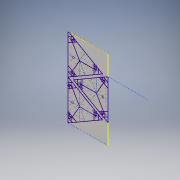
# Autodesk Inventor part: design(60,60,60)_3frames
Saved by Autodesk Inventor 2016 (Build 200138000, 138)
## iProperties
Created: 2016-02-28
Part Number: design(60,60,60)_3frames
Material: Generic
Document SubType Name: Modeling
Designer: Raghu Velagala
Density: 1 g/cm^3
Appearance: Default
Author: Raghu Velagala
Autodesk Inventor part; units mm, degrees
ref_plane "YZ Plane" through (0, 0, 0) normal (1, 0, 0) x (0, 1, 0)
ref_plane "XZ Plane" through (0, 0, 0) normal (0, 1, 0) x (-1, 0, 0)
ref_plane "XY Plane" through (0, 0, 0) normal (0, 0, 1) x (1, 0, 0)
sketch "Sketch1" plane through (0, 0, 0) normal (0, 0, 1) x (1, 0, 0)
  line L0 (0, 0) -> (304.8, 0)
  line L1 (304.8, 0) -> (304.8, 609.6)
  line L2 (304.8, 609.6) -> (0, 609.6)
  line L3 (0, 609.6) -> (0, 0)
  dimension "d4" = 609.6
  dimension "d5" = 304.8
  constraints: 8 end point, 2 parallel, 1 horizontal, 1 perpendicular
  measures "d4" distance of L0.end L1.end
  measures "d5" distance of L1.end L2.end
extrude "Extrusion1" add sketch "Sketch1" along normal blind 1.6002
sketch "3 frames" plane through (0, 0, 1.6002) normal (0, 0, 1) x (1, 0, 0)
  line L0 (0, 609.6) -> (0, 0) projected
  line L1 (0, 609.6) -> (263.9645, 457.2)
  line L2 (0, 609.6) -> (304.8, 609.6) construction
  line L3 (263.9645, 457.2) -> (0, 304.8)
  line L4 (0, 0) -> (263.9645, 152.4)
  line L5 (0, 0) -> (304.8, 0) construction
  line L6 (263.9645, 152.4) -> (0, 304.8)
  line L7 (197.9734, 419.1) -> (197.9734, 495.3)
  line L8 (304.8, 0) -> (304.8, 609.6) projected
  line L9 (304.8, 0) -> (304.8, 609.6) projected
  line L10 (304.8, 459.0878) -> (40.8355, 306.6878)
  line L11 (304.8, 459.0878) -> (609.6, 459.0878) construction
  line L12 (40.8355, 306.6878) -> (304.8, 154.2878)
  line L13 (65.9911, 38.1) -> (0, 76.2)
  line L14 (197.9734, 114.3) -> (197.9734, 190.5)
  line L15 (0, 228.6) -> (65.9911, 266.7)
  line L16 (238.8089, 192.3878) -> (304.8, 230.4878)
  line L17 (238.8089, 420.9878) -> (304.8, 382.8878)
  line L18 (106.8266, 268.5878) -> (106.8266, 344.7878)
  line L19 (65.9911, 342.9) -> (0, 381)
  line L20 (0, 533.4) -> (65.9911, 571.5)
  line L21 (271.8044, 440.0378) -> (304.8, 420.9878)
  line L22 (256.5553, 417.5255) -> (265.1553, 432.4212)
  line L23 (100.9518, 285.6878) -> (83.7518, 285.6878)
  line L24 (256.5553, 195.8501) -> (265.1553, 180.9545)
  line L25 (11.8716, 242.2377) -> (3.2716, 257.1333)
  line L26 (203.8482, 173.4) -> (221.0482, 173.4)
  line L27 (11.8716, 62.5623) -> (3.2716, 47.6667)
  line L28 (203.8482, 478.2) -> (221.0482, 478.2)
  line L29 (48.2447, 568.0377) -> (39.6447, 582.9333)
  line L30 (48.2447, 346.3623) -> (39.6447, 331.4667)
  line L31 (230.969, 133.35) -> (230.969, 171.45)
  line L32 (0, 266.7) -> (32.9956, 285.75)
  line L33 (32.9956, 19.05) -> (0, 38.1)
  line L34 (271.8044, 173.3378) -> (304.8, 192.3878)
  line L35 (73.831, 287.6378) -> (73.831, 325.7378)
  line L36 (0, 342.9) -> (32.9956, 323.85)
  line L37 (230.969, 438.15) -> (230.969, 476.25)
  line L38 (0, 571.5) -> (32.9956, 590.55)
  line L39 (7.5716, 55.1145) -> (25.7582, 44.6145)
  line L40 (212.4482, 173.4) -> (212.4482, 152.4)
  line L41 (7.5716, 249.6855) -> (25.7582, 260.1855)
  line L42 (260.8553, 188.4023) -> (279.0418, 198.9023)
  line L43 (92.3518, 285.6878) -> (92.3518, 306.6878)
  line L44 (260.8553, 424.9733) -> (279.0418, 414.4733)
  line L45 (43.9447, 338.9145) -> (25.7582, 349.4145)
  line L46 (212.4482, 478.2) -> (212.4482, 457.2)
  line L47 (43.9447, 575.4855) -> (25.7582, 564.9855)
  line L48 (0, 304.8) -> (0, 0)
  line L49 (0, 152.4) -> (263.9645, 152.4) construction
  line L50 (0, 304.8) -> (131.9823, 76.2) construction
  line L51 (0, 0) -> (131.9823, 228.6) construction
  line L52 (87.9882, 152.4) -> (87.9882, 45.6952) construction
  line L53 (87.9882, 152.4) -> (87.9882, 254) construction
  line L54 (87.9882, 152.4) -> (25.7582, 260.1855)
  line L55 (87.9882, 152.4) -> (25.7582, 44.6145)
  line L56 (87.9882, 152.4) -> (212.4482, 152.4)
  line L57 (304.8, 459.0878) -> (304.8, 154.2878)
  line L58 (304.8, 459.0878) -> (172.8177, 230.4878) construction
  line L59 (172.8177, 382.8878) -> (304.8, 154.2878) construction
  line L60 (304.8, 306.6878) -> (40.8355, 306.6878) construction
  line L61 (216.8118, 306.6878) -> (216.8118, 408.2878) construction
  line L62 (216.8118, 306.6878) -> (279.0418, 414.4733)
  line L63 (216.8118, 306.6878) -> (279.0418, 198.9023)
  line L64 (216.8118, 306.6878) -> (92.3518, 306.6878)
  line L65 (0, 304.8) -> (0, 609.6)
  line L66 (0, 304.8) -> (131.9823, 533.4) construction
  line L67 (304.8, 609.6) -> (0, 609.6) projected
  line L68 (0, 609.6) -> (131.9823, 381) construction
  line L69 (0, 457.2) -> (263.9645, 457.2) construction
  line L70 (87.9882, 457.2) -> (87.9882, 355.6) construction
  line L71 (87.9882, 457.2) -> (25.7582, 564.9855)
  line L72 (87.9882, 457.2) -> (25.7582, 349.4145)
  line L73 (87.9882, 457.2) -> (212.4482, 457.2)
  point P0 (15.3659, 50.6145)
  point P1 (212.4482, 164.4)
  point P2 (15.3659, 254.1855)
  point P3 (268.6495, 192.9023)
  point P4 (92.3518, 294.6878)
  point P5 (268.6495, 420.4733)
  point P6 (36.1505, 343.4145)
  point P7 (212.4482, 469.2)
  point P8 (36.1505, 570.9855)
  dimension "d7" = 30
  dimension "d9" = 60
  dimension "d11" = 30
  dimension "d20" = 60
  dimension "d27" = 304.8
  dimension "d28" = 150
  dimension "d29" = 304.8
  dimension "d30" = 60
  dimension "d31" = 76.2
  dimension "d32" = 76.2
  dimension "d33" = 76.2
  dimension "d34" = 76.2
  dimension "d35" = 76.2
  dimension "d36" = 76.2
  dimension "d38" = 76.2
  dimension "d39" = 76.2
  dimension "d40" = 76.2
  dimension "d81" = 17.2
  dimension "d82" = 154.2878
  dimension "d83" = 17.2
  dimension "d84" = 17.2
  dimension "d85" = 17.2
  dimension "d86" = 17.2
  dimension "d87" = 17.2
  dimension "d88" = 17.2
  dimension "d89" = 17.2
  dimension "d90" = 17.2
  dimension "d91" = 38.1
  dimension "d118" = 38.1
  dimension "d119" = 38.1
  dimension "d120" = 38.1
  dimension "d121" = 38.1
  dimension "d122" = 38.1
  dimension "d123" = 38.1
  dimension "d124" = 38.1
  dimension "d125" = 38.1
  dimension "d155" = 21
  dimension "d157" = 9
  dimension "d158" = 21
  dimension "d159" = 9
  dimension "d160" = 21
  dimension "d164" = 9
  dimension "d165" = 21
  dimension "d166" = 9
  dimension "d167" = 21
  dimension "d168" = 9
  dimension "d169" = 21
  dimension "d170" = 9
  dimension "d171" = 21
  dimension "d172" = 9
  dimension "d173" = 21
  dimension "d174" = 9
  dimension "d175" = 21
  dimension "d176" = 9
  dimension "d214" = 150
  dimension "d215" = 124.46
  dimension "d216" = 30
  dimension "d217" = 124.46
  dimension "d218" = 124.46
  dimension "d219" = 90
  dimension "d220" = 124.46
  dimension "d221" = 124.46
  dimension "d222" = 124.46
  dimension "d224" = 30
  constraints: 140 end point, 47 point on line, 27 coincident, 18 midpoint, 18 parallel, 17 perpendicular, 4 vertical, 3 equal length, 3 horizontal, 1 collinear, 9 other
  measures "d7" angle of L1 L2
  measures "d9" angle of L1 L3
  measures "d11" angle of L5 L4
  measures "d20" angle of L4 L6
  measures "d27" distance of L10.start L10.end
  measures "d28" angle of L10 L11
  measures "d29" distance of L10.end L12.end
  measures "d30" angle of L12 L10
  measures "d31" distance of L20.start L20.end
  measures "d32" distance of L7.start L7.end
  measures "d33" distance of L19.start L19.end
  measures "d34" distance of L15.start L15.end
  measures "d35" distance of L14.start L14.end
  measures "d36" distance of L18.start L18.end
  measures "d38" distance of L17.start L17.end
  measures "d39" distance of L16.start L16.end
  measures "d40" distance of L13.start L13.end
  measures "d81" distance of L22.start L22.end
  measures "d82" distance of L5.end L12.end
  measures "d83" distance of L23.start L23.end
  measures "d84" distance of L24.start L24.end
  measures "d85" distance of L25.start L25.end
  measures "d86" distance of L26.start L26.end
  measures "d87" distance of L27.start L27.end
  measures "d88" distance of L28.start L28.end
  measures "d89" distance of L29.start L29.end
  measures "d90" distance of L30.start L30.end
  measures "d91" distance of L21.start L21.end
  measures "d118" distance of L31.start L31.end
  measures "d119" distance of L33.start L33.end
  measures "d120" distance of L32.start L32.end
  measures "d121" distance of L34.start L34.end
  measures "d122" distance of L35.start L35.end
  measures "d123" distance of L37.start L37.end
  measures "d124" distance of L36.start L36.end
  measures "d125" distance of L38.start L38.end
  measures "d155" distance of L39.start L39.end
  measures "d157" distance of L39.start point (15.366, 50.614)
  measures "d158" distance of L40.start L40.end
  measures "d159" distance of L40.start point (212.448, 164.4)
  measures "d160" distance of L41.start L41.end
  measures "d164" distance of L41.start point (15.366, 254.186)
  measures "d165" distance of L42.start L42.end
  measures "d166" distance of L42.start point (268.65, 192.902)
  measures "d167" distance of L43.start L43.end
  measures "d168" distance of L43.start point (92.352, 294.688)
  measures "d169" distance of L44.start L44.end
  measures "d170" distance of L44.start point (268.65, 420.473)
  measures "d171" distance of L45.start L45.end
  measures "d172" distance of L45.start point (36.15, 343.414)
  measures "d173" distance of L46.start L46.end
  measures "d174" distance of L46.start point (212.448, 469.2)
  measures "d175" distance of L47.start L47.end
  measures "d176" distance of L47.start point (36.15, 570.986)
  measures "d214" angle of L54 L52
  measures "d215" distance of L52.start L54.end
  measures "d216" angle of L55 L52
  measures "d217" distance of L52.start L55.end
  measures "d218" distance of L52.start L56.end
  measures "d219" angle of L56 L52
  measures "d220" distance of L61.start L62.end
  measures "d221" distance of L61.start L63.end
  measures "d222" distance of L61.start L64.end
  measures "d224" angle of L62 L61
sketch "Holes" plane through (0, 0, 1.6002) normal (0, 0, 1) x (1, 0, 0)
  line L0 (182.8074, 366.1889) -> (205.8074, 366.1889)
  line L1 (205.8074, 366.1889) -> (205.8074, 308.1889)
  line L2 (205.8074, 308.1889) -> (182.8074, 308.1889)
  line L3 (182.8074, 308.1889) -> (182.8074, 366.1889)
  line L4 (102.5125, 80.9532) -> (79.5125, 80.9532)
  line L5 (79.5125, 80.9532) -> (79.5125, 138.9532)
  line L6 (79.5125, 138.9532) -> (102.5125, 138.9532)
  line L7 (102.5125, 138.9532) -> (102.5125, 80.9532)
  line L8 (119.975, 391.4712) -> (96.975, 391.4712)
  line L9 (96.975, 391.4712) -> (96.975, 449.4712)
  line L10 (96.975, 449.4712) -> (119.975, 449.4712)
  line L11 (119.975, 449.4712) -> (119.975, 391.4712)
  line L12 (169.2482, 365.9) -> (218.2482, 365.9)
  line L13 (218.2482, 365.9) -> (218.2482, 307.9)
  line L14 (218.2482, 307.9) -> (169.2482, 307.9)
  line L15 (169.2482, 307.9) -> (169.2482, 365.9)
  line L16 (65.4689, 138.9625) -> (114.4689, 138.9625)
  line L17 (114.4689, 138.9625) -> (114.4689, 80.9625)
  line L18 (114.4689, 80.9625) -> (65.4689, 80.9625)
  line L19 (65.4689, 80.9625) -> (65.4689, 138.9625)
  line L20 (81.5247, 449.4098) -> (130.5247, 449.4098)
  line L21 (130.5247, 449.4098) -> (130.5247, 391.4098)
  line L22 (130.5247, 391.4098) -> (81.5247, 391.4098)
  line L23 (81.5247, 391.4098) -> (81.5247, 449.4098)
  line L24 (285.6758, 284.9583) -> (249.6758, 284.9583)
  line L25 (249.6758, 284.9583) -> (249.6758, 248.9583)
  line L26 (249.6758, 248.9583) -> (285.6758, 248.9583)
  line L27 (285.6758, 248.9583) -> (285.6758, 284.9583)
  line L28 (14.9019, 211.0048) -> (50.9019, 211.0048)
  line L29 (50.9019, 211.0048) -> (50.9019, 175.0048)
  line L30 (50.9019, 175.0048) -> (14.9019, 175.0048)
  line L31 (14.9019, 175.0048) -> (14.9019, 211.0048)
  line L32 (23.8253, 509.4883) -> (59.8253, 509.4883)
  line L33 (59.8253, 509.4883) -> (59.8253, 473.4883)
  line L34 (59.8253, 473.4883) -> (23.8253, 473.4883)
  line L35 (23.8253, 473.4883) -> (23.8253, 509.4883)
  line L36 (91.783, 178.2654) -> (115.783, 178.2654)
  line L37 (115.783, 178.2654) -> (115.783, 209.2654)
  line L38 (115.783, 209.2654) -> (91.783, 209.2654)
  line L39 (91.783, 209.2654) -> (91.783, 178.2654)
  line L40 (199.4394, 276.8758) -> (175.4394, 276.8758)
  line L41 (175.4394, 276.8758) -> (175.4394, 245.8758)
  line L42 (175.4394, 245.8758) -> (199.4394, 245.8758)
  line L43 (199.4394, 245.8758) -> (199.4394, 276.8758)
  line L44 (102.016, 482.8121) -> (126.016, 482.8121)
  line L45 (126.016, 482.8121) -> (126.016, 513.8121)
  line L46 (126.016, 513.8121) -> (102.016, 513.8121)
  line L47 (102.016, 513.8121) -> (102.016, 482.8121)
  line L48 (117.0125, 323.6811) -> (153.0125, 323.6811)
  line L49 (153.0125, 323.6811) -> (153.0125, 287.6811)
  line L50 (153.0125, 287.6811) -> (117.0125, 287.6811)
  line L51 (117.0125, 287.6811) -> (117.0125, 323.6811)
  line L52 (249.6758, 369.949) -> (285.6758, 369.949)
  line L53 (285.6758, 369.949) -> (285.6758, 333.949)
  line L54 (285.6758, 333.949) -> (249.6758, 333.949)
  line L55 (249.6758, 333.949) -> (249.6758, 369.949)
  line L56 (149.725, 170.7351) -> (185.725, 170.7351)
  line L57 (185.725, 170.7351) -> (185.725, 134.7351)
  line L58 (185.725, 134.7351) -> (149.725, 134.7351)
  line L59 (149.725, 134.7351) -> (149.725, 170.7351)
  line L60 (17.1827, 129.9204) -> (53.1827, 129.9204)
  line L61 (53.1827, 129.9204) -> (53.1827, 93.9204)
  line L62 (53.1827, 93.9204) -> (17.1827, 93.9204)
  line L63 (17.1827, 93.9204) -> (17.1827, 129.9204)
  line L64 (152.7155, 476.5755) -> (188.7155, 476.5755)
  line L65 (188.7155, 476.5755) -> (188.7155, 440.5755)
  line L66 (188.7155, 440.5755) -> (152.7155, 440.5755)
  line L67 (152.7155, 440.5755) -> (152.7155, 476.5755)
  line L68 (25.2472, 425.0811) -> (61.2472, 425.0811)
  line L69 (61.2472, 425.0811) -> (61.2472, 389.0811)
  line L70 (61.2472, 389.0811) -> (25.2472, 389.0811)
  line L71 (25.2472, 389.0811) -> (25.2472, 425.0811)
  point P0 (0, 0)
  point P1 (39.4323, 453.5435)
  point P2 (268.1368, 306.5537)
  point P3 (34.6418, 152.3907)
  dimension "d41" = 23
  dimension "d42" = 58
  dimension "d43" = 23
  dimension "d44" = 58
  dimension "d45" = 23
  dimension "d46" = 58
  dimension "d47" = 49
  dimension "d48" = 58
  dimension "d49" = 49
  dimension "d50" = 58
  dimension "d51" = 49
  dimension "d52" = 58
  dimension "d53" = 36
  dimension "d54" = 36
  dimension "d55" = 36
  dimension "d56" = 36
  dimension "d57" = 36
  dimension "d58" = 36
  dimension "d61" = 24
  dimension "d62" = 31
  dimension "d63" = 24
  dimension "d64" = 31
  dimension "d65" = 24
  dimension "d66" = 31
  dimension "d106" = 36
  dimension "d107" = 36
  dimension "d108" = 36
  dimension "d109" = 36
  dimension "d110" = 36
  dimension "d111" = 36
  dimension "d112" = 36
  dimension "d113" = 36
  dimension "d114" = 36
  dimension "d115" = 36
  dimension "d116" = 36
  dimension "d117" = 36
  constraints: 144 end point, 72 coincident, 36 parallel, 18 horizontal, 18 perpendicular
  measures "d41" distance of L1.end L2.end
  measures "d42" distance of L0.end L1.end
  measures "d43" distance of L5.end L6.end
  measures "d44" distance of L4.end L5.end
  measures "d45" distance of L9.end L10.end
  measures "d46" distance of L8.end L9.end
  measures "d47" distance of L13.end L14.end
  measures "d48" distance of L12.end L13.end
  measures "d49" distance of L17.end L18.end
  measures "d50" distance of L16.end L17.end
  measures "d51" distance of L21.end L22.end
  measures "d52" distance of L20.end L21.end
  measures "d53" distance of L26.end L25.end
  measures "d54" distance of L25.end L24.end
  measures "d55" distance of L29.end L30.end
  measures "d56" distance of L28.end L29.end
  measures "d57" distance of L33.end L34.end
  measures "d58" distance of L32.end L33.end
  measures "d61" distance of L38.end L37.end
  measures "d62" distance of L37.end L36.end
  measures "d63" distance of L42.end L41.end
  measures "d64" distance of L41.end L40.end
  measures "d65" distance of L46.end L45.end
  measures "d66" distance of L45.end L44.end
  measures "d106" distance of L49.end L50.end
  measures "d107" distance of L48.end L49.end
  measures "d108" distance of L53.end L54.end
  measures "d109" distance of L52.end L53.end
  measures "d110" distance of L57.end L58.end
  measures "d111" distance of L56.end L57.end
  measures "d112" distance of L61.end L62.end
  measures "d113" distance of L60.end L61.end
  measures "d114" distance of L65.end L66.end
  measures "d115" distance of L64.end L65.end
  measures "d116" distance of L69.end L70.end
  measures "d117" distance of L68.end L69.end
hole "Top Mount Holes" at (96.975, 449.4712, 1.6002) at (119.975, 449.4712, 1.6002) at (96.975, 391.4712, 1.6002) at (119.975, 391.4712, 1.6002) at (81.5247, 449.4098, 1.6002) at (81.5247, 391.4098, 1.6002) at (130.5247, 391.4098, 1.6002) at (130.5247, 449.4098, 1.6002) at (182.8074, 366.1889, 1.6002) at (205.8074, 366.1889, 1.6002) at (218.2482, 365.9, 1.6002) at (218.2482, 307.9, 1.6002) at (169.2482, 307.9, 1.6002) at (169.2482, 365.9, 1.6002) at (114.4689, 138.9625, 1.6002) at (114.4689, 80.9625, 1.6002) at (65.4689, 80.9625, 1.6002) at (65.4689, 138.9625, 1.6002) at (79.5125, 138.9532, 1.6002) at (102.5125, 138.9532, 1.6002) at (102.5125, 80.9532, 1.6002) at (79.5125, 80.9532, 1.6002) at (23.8253, 509.4883, 1.6002) at (59.8253, 509.4883, 1.6002) at (23.8253, 473.4883, 1.6002) at (59.8253, 473.4883, 1.6002) at (249.6758, 284.9583, 1.6002) at (285.6758, 284.9583, 1.6002) at (249.6758, 248.9583, 1.6002) at (285.6758, 248.9583, 1.6002) at (14.9019, 211.0048, 1.6002) at (50.9019, 211.0048, 1.6002) at (50.9019, 175.0048, 1.6002) at (14.9019, 175.0048, 1.6002) at (175.4394, 276.8758, 1.6002) at (199.4394, 276.8758, 1.6002) at (175.4394, 245.8758, 1.6002) at (199.4394, 245.8758, 1.6002) at (126.016, 482.8121, 1.6002) at (102.016, 482.8121, 1.6002) at (91.783, 209.2654, 1.6002) at (115.783, 209.2654, 1.6002) at (126.016, 513.8121, 1.6002) at (102.016, 513.8121, 1.6002) at (115.783, 178.2654, 1.6002) at (91.783, 178.2654, 1.6002) at (205.8074, 308.1889, 1.6002) at (182.8074, 308.1889, 1.6002) at (117.0125, 323.6811, 1.6002) at (153.0125, 323.6811, 1.6002) direction (0, 0, -1) diameter 2.5 end through all and at (117.0125, 287.6811, 1.6002) (153.0125, 287.6811, 1.6002) (249.6758, 369.949, 1.6002) (285.6758, 369.949, 1.6002) (249.6758, 333.949, 1.6002) (285.6758, 333.949, 1.6002) (53.1827, 129.9204, 1.6002) (17.1827, 129.9204, 1.6002) (17.1827, 93.9204, 1.6002) (53.1827, 93.9204, 1.6002) (149.725, 170.7351, 1.6002) (185.725, 170.7351, 1.6002) (185.725, 134.7351, 1.6002) (149.725, 134.7351, 1.6002) (61.2472, 389.0811, 1.6002) (25.2472, 389.0811, 1.6002) (25.2472, 425.0811, 1.6002) (61.2472, 425.0811, 1.6002) (188.7155, 476.5755, 1.6002) (152.7155, 476.5755, 1.6002) (152.7155, 440.5755, 1.6002) (188.7155, 440.5755, 1.6002)
hole "Wire-through Holes" at (39.4323, 453.5435, 1.6002) at (268.1368, 306.5537, 1.6002) at (34.6418, 152.3907, 1.6002) direction (0, 0, -1) diameter 18 end through all
hole "Motor Mount Holes" at (48.2447, 568.0377, 1.6002) at (39.6447, 582.9333, 1.6002) at (221.0482, 478.2, 1.6002) at (203.8482, 478.2, 1.6002) at (48.2447, 346.3623, 1.6002) at (39.6447, 331.4667, 1.6002) at (256.5553, 417.5255, 1.6002) at (265.1553, 432.4212, 1.6002) at (100.9518, 285.6878, 1.6002) at (83.7518, 285.6878, 1.6002) at (265.1553, 180.9545, 1.6002) at (256.5553, 195.8501, 1.6002) at (11.8716, 242.2377, 1.6002) at (3.2716, 257.1333, 1.6002) at (221.0482, 173.4, 1.6002) at (203.8482, 173.4, 1.6002) at (3.2716, 47.6667, 1.6002) at (11.8716, 62.5623, 1.6002) at (265.1553, 432.4212, 1.6002) at (256.5553, 417.5255, 1.6002) direction (0, 0, -1) diameter 2.5 end through all
hole "Motor Axle Holes" at (25.7582, 44.6145, 1.6002) at (25.7582, 260.1855, 1.6002) at (212.4482, 152.4, 1.6002) at (279.0418, 198.9023, 1.6002) at (92.3518, 306.6878, 1.6002) at (25.7582, 349.4145, 1.6002) at (279.0418, 414.4733, 1.6002) at (212.4482, 457.2, 1.6002) at (25.7582, 564.9855, 1.6002) direction (0, 0, -1) diameter 17 end through all
hole "Motor Pro. Holes" at (15.3659, 50.6145, 1.6002) at (212.4482, 164.4, 1.6002) at (268.6495, 192.9023, 1.6002) at (92.3518, 294.6878, 1.6002) at (15.3659, 254.1855, 1.6002) at (36.1505, 343.4145, 1.6002) at (268.6495, 420.4733, 1.6002) at (212.4482, 469.2, 1.6002) at (36.1505, 570.9855, 1.6002) direction (0, 0, -1) diameter 2.5 end through all
body "Solid1"
